Autodesk Inventor part; units mm, degrees
(part 7 of 7)
sketch "Dach bez graweru" plane through (0, 0, 2) normal (0, 0, 1) x (1, 0, 0)
  circle A0 centre (-9.75, -51.55) radius 1.5 projected
  circle A1 centre (3.25, -51.55) radius 1.5 projected
  circle A2 centre (3.25, -45.05) radius 1.5 projected
  circle A3 centre (3.25, 6.65) radius 1.5 projected
  circle A4 centre (3.25, 13.15) radius 1.5 projected
  circle A5 centre (-9.75, 13.15) radius 1.5 projected
  circle A6 centre (-67.4121, -60.2) radius 1.5 projected
  circle A7 centre (-74.1621, -60.2) radius 1.5 projected
  circle A8 centre (-67.4121, 21.8) radius 1.5 projected
  circle A9 centre (-74.1621, 21.8) radius 1.5 projected
  arc A10 (-41.8371, -69.2) -> (-41.3371, -68.7) centre (-41.8371, -68.7) ccw projected
  line L0 (-78.3805, -69.2) -> (-41.8371, -69.2) projected
  line L1 (-78.3805, 30.8) -> (-78.3805, -69.2) projected
  line L2 (-41.8371, 30.8) -> (-78.3805, 30.8) projected
  arc A11 (-41.3371, 30.3) -> (-41.8371, 30.8) centre (-41.8371, 30.3) ccw projected
  line L3 (-41.3371, 11.3) -> (-41.3371, 30.3) projected
  line L4 (-13, 11.3) -> (-41.3371, 11.3) projected
  line L5 (-13, 17) -> (-13, 11.3) projected
  line L6 (6.3, 17) -> (-13, 17) projected
  line L7 (6.3, -55.4) -> (6.3, 17) projected
  line L8 (-13, -55.4) -> (6.3, -55.4) projected
  line L9 (-13, -49.7) -> (-13, -55.4) projected
  line L10 (-41.3371, -49.7) -> (-13, -49.7) projected
  line L11 (-41.3371, -68.7) -> (-41.3371, -49.7) projected
  arc A12 (-43.494, 4.7213) -> (-43.9933, 4.2482) centre (-43.494, 4.2213) ccw projected
  line L12 (-38.269, 4.7213) -> (-43.494, 4.7213) projected
  arc A13 (-38.269, 4.7213) -> (-37.769, 5.2213) centre (-38.269, 5.2213) ccw projected
  line L13 (-37.769, 7.1787) -> (-37.769, 5.2213) projected
  arc A14 (-37.769, 7.1787) -> (-38.269, 7.6787) centre (-38.269, 7.1787) ccw projected
  line L14 (-43.494, 7.6787) -> (-38.269, 7.6787) projected
  arc A15 (-43.994, 8.1787) -> (-43.494, 7.6787) centre (-43.494, 8.1787) ccw projected
  line L15 (-43.994, 9.275) -> (-43.994, 8.1787) projected
  arc A16 (-43.994, 9.275) -> (-44.494, 9.775) centre (-44.494, 9.275) ccw projected
  line L16 (-49.494, 9.775) -> (-44.494, 9.775) projected
  arc A17 (-49.494, 9.775) -> (-49.994, 9.275) centre (-49.494, 9.275) ccw projected
  line L17 (-49.994, 4.275) -> (-49.994, 9.275) projected
  arc A18 (-49.994, 4.275) -> (-49.494, 3.775) centre (-49.494, 4.275) ccw projected
  line L18 (-44.4926, 3.775) -> (-49.494, 3.775) projected
  arc A19 (-44.4926, 3.775) -> (-43.9933, 4.2482) centre (-44.4926, 4.275) ccw projected
  line L19 (-15.8027, -38.1) -> (-15.8027, -0.3) projected
  line L20 (-1.0973, -38.6) -> (-15.3027, -38.6) projected
  line L21 (-0.5973, -0.3) -> (-0.5973, -38.1) projected
  line L22 (-15.3027, 0.2) -> (-1.0973, 0.2) projected
  line L23 (-42.0344, -38.6) -> (-56.2398, -38.6) projected
  line L24 (-41.5344, -0.3) -> (-41.5344, -38.1) projected
  line L25 (-56.2398, 0.2) -> (-42.0344, 0.2) projected
  line L26 (-56.7398, -38.1) -> (-56.7398, -0.3) projected
  line L27 (-13.5155, 5.8092) -> (-8.3155, 5.8092) projected
  line L28 (-13.5155, 0.6092) -> (-13.5155, 5.8092) projected
  line L29 (-8.3155, 0.6092) -> (-13.5155, 0.6092) projected
  line L30 (-8.3155, 5.8092) -> (-8.3155, 0.6092) projected
  line L31 (-21.4873, -42.1072) -> (-16.2873, -42.1072) projected
  line L32 (-21.4873, -47.3072) -> (-21.4873, -42.1072) projected
  line L33 (-16.2873, -47.3072) -> (-21.4873, -47.3072) projected
  line L34 (-16.2873, -42.1072) -> (-16.2873, -47.3072) projected
  circle A20 centre (-17.024, 4.925) radius 1 projected
  arc A21 (-34.5609, -6.5715) -> (-34.319, -6.1433) centre (-34.819, -6.1433) ccw projected
  arc A22 (-34.5609, -6.5715) -> (-34.8027, -6.9997) centre (-34.3027, -6.9997) ccw projected
  line L35 (-34.8027, -31.5) -> (-34.8027, -6.9997) projected
  line L36 (-28.019, -31.5) -> (-34.8027, -31.5) projected
  arc A23 (-27.519, -32) -> (-28.019, -31.5) centre (-28.019, -32) ccw projected
  line L37 (-27.519, -37.725) -> (-27.519, -32) projected
  arc A24 (-28.019, -38.225) -> (-27.519, -37.725) centre (-28.019, -37.725) ccw projected
  line L38 (-32.144, -38.225) -> (-28.019, -38.225) projected
  line L39 (-32.144, -47.7) -> (-32.144, -38.225) projected
  line L40 (-27.144, -47.7) -> (-32.144, -47.7) projected
  line L41 (-27.144, -40.025) -> (-27.144, -47.7) projected
  arc A25 (-26.644, -39.525) -> (-27.144, -40.025) centre (-26.644, -40.025) ccw projected
  line L42 (-23.519, -39.525) -> (-26.644, -39.525) projected
  arc A26 (-23.519, -39.525) -> (-23.019, -39.025) centre (-23.519, -39.025) ccw projected
  line L43 (-23.019, -32) -> (-23.019, -39.025) projected
  arc A27 (-22.519, -31.5) -> (-23.019, -32) centre (-22.519, -32) ccw projected
  line L44 (-17.8027, -31.5) -> (-22.519, -31.5) projected
  line L45 (-17.8027, -6.5) -> (-17.8027, -31.5) projected
  line L46 (-20.369, -6.5) -> (-17.8027, -6.5) projected
  arc A28 (-20.869, -6) -> (-20.369, -6.5) centre (-20.369, -6) ccw projected
  line L47 (-20.869, 1.075) -> (-20.869, -6) projected
  arc A29 (-20.869, 1.075) -> (-21.369, 1.575) centre (-21.369, 1.075) ccw projected
  line L48 (-22.9273, 1.575) -> (-21.369, 1.575) projected
  arc A30 (-23.3621, 2.3219) -> (-22.9273, 1.575) centre (-22.9273, 2.075) ccw projected
  arc A31 (-23.3621, 2.3219) -> (-31.4585, 2.8843) centre (-27.2755, 4.5435) ccw projected
  arc A32 (-31.9232, 2.2) -> (-31.4585, 2.8843) centre (-31.9232, 2.7) ccw projected
  line L49 (-33.819, 2.2) -> (-31.9232, 2.2) projected
  arc A33 (-33.819, 2.2) -> (-34.319, 1.7) centre (-33.819, 1.7) ccw projected
  line L50 (-34.319, -6.1433) -> (-34.319, 1.7) projected
  arc A34 (-15.3027, 0.2) -> (-15.8027, -0.3) centre (-15.3027, -0.3) ccw projected
  arc A35 (-15.8027, -38.1) -> (-15.3027, -38.6) centre (-15.3027, -38.1) ccw projected
  arc A36 (-1.0973, -38.6) -> (-0.5973, -38.1) centre (-1.0973, -38.1) ccw projected
  arc A37 (-0.5973, -0.3) -> (-1.0973, 0.2) centre (-1.0973, -0.3) ccw projected
  arc A38 (-56.2398, 0.2) -> (-56.7398, -0.3) centre (-56.2398, -0.3) ccw projected
  arc A39 (-56.7398, -38.1) -> (-56.2398, -38.6) centre (-56.2398, -38.1) ccw projected
  arc A40 (-42.0344, -38.6) -> (-41.5344, -38.1) centre (-42.0344, -38.1) ccw projected
  arc A41 (-41.5344, -0.3) -> (-42.0344, 0.2) centre (-42.0344, -0.3) ccw projected
  point P0 (0, 0)
sketch "Sketch8" plane through (0, 0, 2) normal (0, 0, 1) x (1, 0, 0)
  line L0 (-46.732, -41.2252) -> (-46.732, -62.1936) construction
  line L1 (-46.732, -62.1936) -> (-55.4995, -62.1936) construction
  line L2 (-55.4995, -62.1936) -> (-55.4995, -41.2252) construction
  line L3 (-55.4995, -41.2252) -> (-46.732, -41.2252) construction
  point P0 (0, 0)
  constraints: 2 other
extrude "Extrusion5" [suppressed]
equation "\"d15\" = d14"
equation "\"d27\" = d26"
equation "\"d28\" = d24"
equation "\"d29\" = d26"
equation "\"d30\" = d26"
equation "\"d32\" = d24"
equation "\"d33\" = d26"
equation "\"d34\" = d26"
equation "\"d42\" = d41"
equation "\"d44\" = d41"
equation "\"d46\" = d45"
body "Solid1"
